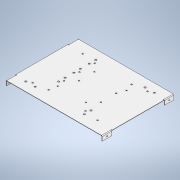
# Autodesk Inventor part: soporte_resistencias
Saved by Autodesk Inventor 2021 (Build 250183000, 183)
## iProperties
Created: 2021-04-16
Part Number: soporte_resistencias
Material: Acero ASTM A36
Document SubType Name: Chapa
Designer: Leonardo Fabio Mercado Benítez
Density: 7.85 g/cm^3
Sheet Metal Rule: Por defecto_mm
Appearance: Placa
Author: Leonardo Fabio Mercado Benítez
Autodesk Inventor part; units mm, degrees
ref_plane "YZ Plane" through (0, 0, 0) normal (1, 0, 0) x (0, 1, 0)
ref_plane "XZ Plane" through (0, 0, 0) normal (0, 1, 0) x (-1, 0, 0)
ref_plane "XY Plane" through (0, 0, 0) normal (0, 0, 1) x (1, 0, 0)
sketch "Boceto1" plane through (0, 0, 0) normal (0, 1, 0) x (-1, 0, 0)
  line L0 (255.94, 190.94) -> (-255.94, 190.94)
  line L1 (-255.94, 190.94) -> (-255.94, -190.94)
  line L2 (-255.94, -190.94) -> (255.94, -190.94)
  line L3 (255.94, -190.94) -> (255.94, 190.94)
  line L4 (255.94, 190.94) -> (-255.94, -190.94) construction
  line L5 (-255.94, 190.94) -> (255.94, -190.94) construction
  point P0 (0, 0)
  dimension "d0" = 511.88
  dimension "d1" = 381.88
  measures "d0" distance of L2.end L1.end
  measures "d1" distance of L1.end L0.end
extrude "Placa1" add sketch "Boceto1" along normal blind 1.9
sketch "Boceto3" plane through (0, 1.9, 0) normal (0, 1, 0) x (1, 0, 0)
  circle A0 centre (172.5, 133.66) radius 3.675
  circle A1 centre (172.5, -132.34) radius 3.675
  circle A2 centre (98, 123.16) radius 3.675
  circle A3 centre (98, 41.49) radius 3.675
  circle A4 centre (98, -40.17) radius 3.675
  circle A5 centre (98, -121.84) radius 3.675
  circle A6 centre (-98, 123.16) radius 3.675
  circle A7 centre (-98, 41.49) radius 3.675
  circle A8 centre (-98, -40.17) radius 3.675
  circle A9 centre (-98, -121.84) radius 3.675
  circle A10 centre (-172.5, 133.66) radius 3.675
  circle A11 centre (-172.5, -132.34) radius 3.675
  point P0 (0, 0)
  dimension "d13" = 7.35
  dimension "d14" = 7.35
  dimension "d15" = 7.35
  dimension "d16" = 7.35
  dimension "d17" = 7.35
  dimension "d18" = 7.35
  dimension "d19" = 7.35
  dimension "d20" = 7.35
  dimension "d21" = 7.35
  dimension "d22" = 7.35
  dimension "d23" = 7.35
  dimension "d24" = 7.35
  constraints: 12 centre point
  measures "d13" diameter of A0
  measures "d14" diameter of A1
  measures "d15" diameter of A2
  measures "d16" diameter of A3
  measures "d17" diameter of A4
  measures "d18" diameter of A5
  measures "d19" diameter of A6
  measures "d20" diameter of A7
  measures "d21" diameter of A8
  measures "d22" diameter of A9
  measures "d23" diameter of A10
  measures "d24" diameter of A11
extrude "Cortar1" cut sketch "Boceto3" against normal blind 1.9
sketch "Boceto4" plane through (0, 1.9, 0) normal (0, 1, 0) x (1, 0, 0)
  circle A0 centre (-197.5, -144.14) radius 4.7625
  circle A1 centre (-147.5, -144.14) radius 4.7625
  circle A2 centre (-109.8, 140.6937) radius 4.7625
  circle A3 centre (-109.8, 105.671) radius 4.7625
  circle A4 centre (-109.8, 59.0237) radius 4.7625
  circle A5 centre (-109.8, 24.001) radius 4.7625
  circle A6 centre (-109.8, -22.6363) radius 4.7625
  circle A7 centre (-109.8, -57.659) radius 4.7625
  circle A8 centre (147.5, 145.46) radius 4.7625
  circle A9 centre (197.5, 145.46) radius 4.7625
  circle A10 centre (109.8, -104.351) radius 4.7625
  circle A11 centre (109.8, -139.3737) radius 4.7625
  point P0 (0, 0)
  dimension "d27" = 9.525
  dimension "d28" = 9.525
  dimension "d29" = 9.525
  dimension "d30" = 9.525
  dimension "d31" = 9.525
  dimension "d32" = 9.525
  dimension "d33" = 9.525
  dimension "d34" = 9.525
  dimension "d35" = 9.525
  dimension "d36" = 9.525
  dimension "d37" = 9.525
  dimension "d38" = 9.525
  constraints: 12 centre point
  measures "d27" diameter of A0
  measures "d28" diameter of A1
  measures "d29" diameter of A2
  measures "d30" diameter of A3
  measures "d31" diameter of A4
  measures "d32" diameter of A5
  measures "d33" diameter of A6
  measures "d34" diameter of A7
  measures "d35" diameter of A8
  measures "d36" diameter of A9
  measures "d37" diameter of A10
  measures "d38" diameter of A11
extrude "Cortar2" cut sketch "Boceto4" against normal blind 1.9
sketch "Boceto5" plane through (0, 1.9, 0) normal (0, 1, 0) x (1, 0, 0)
  line L0 (-122.5, 88.16) -> (122.5, 88.16) projected
  line L1 (122.5, 76.49) -> (-122.5, 76.49) projected
  line L2 (-122.5, 6.49) -> (122.5, 6.49) projected
  line L3 (122.5, -5.17) -> (-122.5, -5.17) projected
  line L4 (-122.5, -75.17) -> (122.5, -75.17) projected
  line L5 (122.5, -86.84) -> (-122.5, -86.84) projected
  line L6 (-122.5, 76.49) -> (-122.5, 88.16) construction
  line L7 (122.5, 88.16) -> (122.5, 76.49) construction
  line L8 (-122.5, 6.49) -> (-122.5, -5.17) construction
  line L9 (122.5, 6.49) -> (122.5, -5.17) construction
  line L10 (-122.5, -75.17) -> (-122.5, -86.84) construction
  line L11 (122.5, -75.17) -> (122.5, -86.84) construction
  line L12 (-122.5, 82.325) -> (122.5, 82.325) construction
  line L13 (-122.5, 0.66) -> (122.5, 0.66) construction
  line L14 (-122.5, -81.005) -> (122.5, -81.005) construction
  line L15 (-122.5, 82.325) -> (-59, 82.325) construction
  line L16 (-122.5, 0.66) -> (-59, 0.66) construction
  line L17 (122.5, -81.005) -> (59, -81.005) construction
  line L18 (-122.5, -81.005) -> (-90.75, -81.005) construction
  line L19 (122.5, 82.325) -> (112.5, 82.325) construction
  circle A0 centre (-59, 82.325) radius 3.175
  circle A1 centre (112.5, 82.325) radius 3.175
  circle A2 centre (-59, 0.66) radius 3.175
  circle A3 centre (-90.75, -81.005) radius 3.175
  circle A4 centre (59, -81.005) radius 3.175
  point P0 (0, 0)
  dimension "d42" = 63.5
  dimension "d43" = 63.5
  dimension "d44" = 63.5
  dimension "d45" = 31.75
  dimension "d46" = 10
  dimension "d47" = 6.35
  dimension "d48" = 6.35
  dimension "d49" = 6.35
  dimension "d50" = 6.35
  dimension "d51" = 6.35
  constraints: 28 end point, 6 midpoint, 5 centre point, 5 coincident, 5 point on line, 3 parallel, 2 perpendicular, 1 vertical
  measures "d42" distance of L12.start L15.end
  measures "d43" distance of L13.start L16.end
  measures "d44" distance of L14.end L17.end
  measures "d45" distance of L14.start L18.end
  measures "d46" distance of L12.end L19.end
  measures "d47" diameter of A0
  measures "d48" diameter of A1
  measures "d49" diameter of A2
  measures "d50" diameter of A3
  measures "d51" diameter of A4
extrude "Cortar3" cut sketch "Boceto5" against normal blind 1.9
sketch "Boceto6" plane through (255.94, 0, 190.94) normal (1, 0, 0) x (0, 0, -1)
  line L0 (381.88, 1.9) -> (0, 1.9)
  line L1 (0, 1.9) -> (50.8, 1.9)
  line L2 (50.8, 1.9) -> (50.8, -23.5)
  line L3 (50.8, -23.5) -> (0, -23.5)
  line L4 (0, -23.5) -> (0, 1.9)
  line L5 (381.88, 0) -> (381.88, 1.9)
  line L6 (381.88, 1.9) -> (331.08, 1.9)
  line L7 (331.08, 1.9) -> (331.08, -23.5)
  line L8 (331.08, -23.5) -> (381.88, -23.5)
  line L9 (381.88, -23.5) -> (381.88, 1.9)
  point P0 (190.94, 0)
  dimension "d54" = 50.8
  dimension "d55" = 25.4
  dimension "d56" = 50.8
  dimension "d57" = 25.4
  measures "d54" distance of L2.end L3.end
  measures "d55" distance of L1.end L2.end
  measures "d56" distance of L8.end L7.end
  measures "d57" distance of L7.end L6.end
sheet face with bend "Cara2" sketch "Boceto6" thickness 1.9 toward (-1, 0, 0) bend radius 1.9 relief straight relief width 1.9 relief depth 0.95
bend "Doblez2"
sketch "Boceto7" plane through (-255.94, 0, -190.94) normal (-1, 0, 0) x (0, 0, 1)
  line L0 (0, 1.9) -> (0, 0)
  line L1 (0, 1.9) -> (50.8, 1.9)
  line L2 (50.8, 1.9) -> (50.8, -23.5)
  line L3 (50.8, -23.5) -> (0, -23.5)
  line L4 (0, -23.5) -> (0, 1.9)
  line L5 (381.88, 0) -> (381.88, 1.9)
  line L6 (381.88, 1.9) -> (331.08, 1.9)
  line L7 (331.08, 1.9) -> (331.08, -23.5)
  line L8 (331.08, -23.5) -> (381.88, -23.5)
  line L9 (381.88, -23.5) -> (381.88, 1.9)
  point P0 (190.94, 0)
  dimension "d63" = 50.8
  dimension "d64" = 25.4
  dimension "d65" = 50.8
  dimension "d66" = 25.4
  measures "d63" distance of L2.end L3.end
  measures "d64" distance of L1.end L2.end
  measures "d65" distance of L8.end L7.end
  measures "d66" distance of L7.end L6.end
sheet face with bend "Cara3" sketch "Boceto7" thickness 1.9 toward (1, 0, 0) bend radius 1.9 relief straight relief width 1.9 relief depth 0.95
bend "Doblez3"
sketch "Boceto8" plane through (-255.94, 0, -190.94) normal (-1, 0, 0) x (0, 0, 1)
  line L0 (0, -23.5) -> (0, -1.9) construction
  line L1 (50.8, -1.9) -> (50.8, -23.5) construction
  line L2 (0, -23.5) -> (50.8, -1.9) construction
  line L3 (0, -1.9) -> (50.8, -1.9) construction
  line L4 (0, -1.9) -> (50.8, -23.5) construction
  line L5 (331.08, -1.9) -> (331.08, -23.5) construction
  line L6 (381.88, -1.9) -> (331.08, -1.9) construction
  line L7 (331.08, -23.5) -> (381.88, -1.9) construction
  line L8 (331.08, -1.9) -> (331.08, 0) construction
  line L9 (381.88, -23.5) -> (381.88, -1.9) construction
  line L10 (331.08, -1.9) -> (381.88, -23.5) construction
  circle A0 centre (25.4, -12.7) radius 3.175
  circle A1 centre (356.48, -12.7) radius 3.175
  point P0 (190.94, 0)
  dimension "d72" = 6.35
  dimension "d73" = 6.35
  constraints: 8 end point, 2 centre point, 2 midpoint
  measures "d72" diameter of A0
  measures "d73" diameter of A1
extrude "Extrusión1" cut sketch "Boceto8" against normal up to surface (1.9 mm away)
sketch "Boceto9" plane through (255.94, 0, 190.94) normal (1, 0, 0) x (0, 0, -1)
  line L0 (50.8, -23.5) -> (0, -23.5) construction
  line L1 (50.8, -1.9) -> (0, -1.9) construction
  line L2 (0, -23.5) -> (50.8, -1.9) construction
  line L3 (0, -1.9) -> (50.8, -23.5) construction
  line L4 (381.88, -23.5) -> (331.08, -23.5) construction
  line L5 (381.88, -1.9) -> (381.88, -23.5) construction
  line L6 (331.08, -23.5) -> (381.88, -1.9) construction
  line L7 (331.08, -1.9) -> (381.88, -1.9) construction
  line L8 (331.08, -1.9) -> (381.88, -23.5) construction
  circle A0 centre (25.4, -12.7) radius 3.175
  circle A1 centre (356.48, -12.7) radius 3.175
  point P0 (190.94, 0)
  dimension "d76" = 6.35
  dimension "d77" = 6.35
  constraints: 8 end point, 2 centre point, 2 midpoint
  measures "d76" diameter of A0
  measures "d77" diameter of A1
extrude "Extrusión2" cut sketch "Boceto9" against normal up to surface (1.9 mm away)
equation "\"d25\" = Grosor"
equation "\"d39\" = Grosor"
equation "\"d52\" = Grosor"
equation "\"d2\" = Grosor"
equation "\"d58\" = Radio_pliegue"
equation "\"d59\" = Anchura_desahogo_plegado"
equation "\"d61\" = Remanente_mínimo"
equation "\"Radio_pliegue\" = Grosor"
equation "\"Remanente_mínimo\" = 2 * Grosor"
equation "\"TamañoSeparación\" = Grosor"
equation "\"Radiodetransición\" = Radio_pliegue"
equation "\"Tamaño_destalonado\" = 4 * Grosor"
equation "\"Anchura_desahogo_plegado\" = Grosor"
equation "\"Tamaño_de_radio_de_Jacobi\" = Radio_pliegue"
equation "\"Profundidad_desahogo_plegado\" = 0.5 * Grosor"
equation "\"d60\" = Profundidad_desahogo_plegado"
equation "\"d62\" = Radiodetransición"
equation "\"d67\" = Radio_pliegue"
equation "\"d68\" = Anchura_desahogo_plegado"
equation "\"d70\" = Remanente_mínimo"
equation "\"d69\" = Profundidad_desahogo_plegado"
equation "\"d71\" = Radiodetransición"
equation "\"Grosor\" = 1.9"
